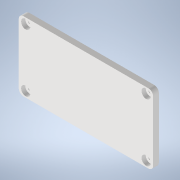
# Autodesk Inventor part: lID
Saved by Autodesk Inventor 2022 (Build 260153000, 153)
## iProperties
Created: 2021-11-08
Part Number: lID
Material: Generisch
Document SubType Name: Modeling
Designer: lukas
Density: 1 g/cm^3
Appearance: Vorgabe
Author: lukas
Autodesk Inventor part; units mm, degrees
ref_plane "YZ Plane" through (0, 0, 0) normal (1, 0, 0) x (0, 1, 0)
ref_plane "XZ Plane" through (0, 0, 0) normal (0, 1, 0) x (-1, 0, 0)
ref_plane "XY Plane" through (0, 0, 0) normal (0, 0, 1) x (1, 0, 0)
sketch "Skizze1" plane through (0, 0, 0) normal (0, 0, 1) x (1, 0, 0)
  arc A0 (-27, 15) -> (-29, 13) centre (-27, 13) ccw projected
  line L0 (-29, 13) -> (-29, 6.9165) projected
  line L1 (-29, 6.9165) -> (-27, 6.9165) projected
  line L2 (-27, 6.9165) -> (-27, 10) projected
  line L3 (-27, 10) -> (-23, 10) projected
  line L4 (-23, 13) -> (-23, 10) projected
  line L5 (-23, 13) -> (23, 13) projected
  line L6 (23, 10) -> (23, 13) projected
  line L7 (27, 10) -> (23, 10) projected
  line L8 (27, 10) -> (27, -10) projected
  line L9 (27, -10) -> (23, -10) projected
  line L10 (23, -13) -> (23, -10) projected
  line L11 (23, -13) -> (-23, -13) projected
  line L12 (-23, -10) -> (-23, -13) projected
  line L13 (-27, -10) -> (-23, -10) projected
  line L14 (-27, -10) -> (-27, -6.9165) projected
  line L15 (-27, -6.9165) -> (-29, -6.9165) projected
  line L16 (-29, -6.9165) -> (-29, -13) projected
  arc A1 (-29, -13) -> (-27, -15) centre (-27, -13) ccw projected
  line L17 (-27, -15) -> (27, -15) projected
  arc A2 (27, -15) -> (29, -13) centre (27, -13) ccw projected
  line L18 (29, -13) -> (29, 13) projected
  arc A3 (29, 13) -> (27, 15) centre (27, 13) ccw projected
  line L19 (27, 15) -> (-27, 15) projected
  circle A4 centre (26, -12.5) radius 1.6 projected
  circle A5 centre (-26, -12.5) radius 1.6 projected
  circle A6 centre (26, 12.5) radius 1.6 projected
  circle A7 centre (-26, 12.5) radius 1.6 projected
  line L20 (-29, 6.9165) -> (-29, -6.9165)
  point P0 (0, 0)
  constraints: 2 end point, 1 collinear
extrude "Extrusion1" add sketch "Skizze1" along normal blind 2.5 contours L19 A3 L18 A2 L17 A1 L16 L15 L14 L13 L12 L11 L10 L9 L8 L7 L6 L5 L4 L3 L2 L1 L0 A0 | L1 L2 L3 L4 L5 L6 L7 L8 L9 L10 L11 L12 L13 L14 L15 L20 | A4 | A5 | A6 | A7
sketch "Skizze2" plane through (0, 0, 2.5) normal (0, 0, 1) x (1, 0, 0)
  circle A0 centre (26, 12.5) radius 1.6 projected
  circle A1 centre (26, -12.5) radius 1.6 projected
  circle A2 centre (-26, -12.5) radius 1.6 projected
  circle A3 centre (-26, 12.5) radius 1.6 projected
  point P0 (0, 0)
hole "Bohrung1" at (-26, -12.5, 2.5) at (-26, 12.5, 2.5) at (26, 12.5, 2.5) at (26, -12.5, 2.5) direction (0, 0, -1) diameter 1.85 end through all counterbore diameter 4 counterbore depth 1.8
sketch "Skizze3" plane through (0, 0, 0) normal (0, 0, -1) x (-1, 0, 0)
  line L0 (12, -13) -> (23, -13) projected
  line L1 (-13, -13) -> (12, -13) projected
  line L2 (-23, -13) -> (-13, -13) projected
  line L3 (23, 13) -> (-23, 13) projected
  line L4 (27, 6.9165) -> (27, 10) projected
  line L5 (27, -10) -> (27, -6.9165) projected
  line L6 (23, -10) -> (23, -13) projected
  line L7 (27, -10) -> (23, -10) projected
  line L8 (-23, -13) -> (-23, -10) projected
  line L9 (-27, -10) -> (-23, -10) projected
  line L10 (23, 13) -> (23, 10) projected
  line L11 (27, 10) -> (23, 10) projected
  line L12 (-23, 10) -> (-23, 13) projected
  line L13 (-27, 10) -> (-23, 10) projected
  line L14 (-27, 10) -> (-27, -10) projected
  line L15 (26.85, 6.9165) -> (26.85, 9.85)
  line L16 (26.85, 9.85) -> (22.85, 9.85)
  line L17 (22.85, 9.85) -> (22.85, 12.85)
  line L18 (22.85, 12.85) -> (-22.85, 12.85)
  line L19 (-22.85, 12.85) -> (-22.85, 9.85)
  line L20 (-22.85, 9.85) -> (-26.85, 9.85)
  line L21 (-26.85, 9.85) -> (-26.85, -9.85)
  line L22 (-26.85, -9.85) -> (-22.85, -9.85)
  line L23 (-22.85, -9.85) -> (-22.85, -12.85)
  line L24 (-22.85, -12.85) -> (-13, -12.85)
  line L25 (-13, -12.85) -> (12, -12.85)
  line L26 (12, -12.85) -> (22.85, -12.85)
  line L27 (22.85, -12.85) -> (22.85, -9.85)
  line L28 (22.85, -9.85) -> (26.85, -9.85)
  line L29 (26.85, -9.85) -> (26.85, -6.9165)
  line L30 (25.85, -6.9165) -> (25.85, -8.85)
  line L31 (25.85, -8.85) -> (21.85, -8.85)
  line L32 (21.85, -8.85) -> (21.85, -11.85)
  line L33 (21.85, -11.85) -> (12, -11.85)
  line L34 (12, -11.85) -> (-13, -11.85)
  line L35 (-13, -11.85) -> (-21.85, -11.85)
  line L36 (-21.85, -11.85) -> (-21.85, -8.85)
  line L37 (-21.85, -8.85) -> (-25.85, -8.85)
  line L38 (-25.85, -8.85) -> (-25.85, 8.85)
  line L39 (-25.85, 8.85) -> (-21.85, 8.85)
  line L40 (-21.85, 8.85) -> (-21.85, 11.85)
  line L41 (-21.85, 11.85) -> (21.85, 11.85)
  line L42 (21.85, 11.85) -> (21.85, 8.85)
  line L43 (21.85, 8.85) -> (25.85, 8.85)
  line L44 (25.85, 8.85) -> (25.85, 6.9165)
  line L45 (26.85, -7.4165) -> (25.8168, -7.4165)
  line L46 (26.85, 7.4165) -> (25.85, 7.4165)
  point P0 (0, 0)
  point P1 (25.85, -7.4165)
  dimension "d9" = 0.15
  dimension "d10" = 1
  dimension "d11" = 0.5
  dimension "d12" = 0.5
  constraints: 64 end point, 3 point on line, 2 horizontal alignment, 2 perpendicular, 28 other
  measures "d9" distance between parallel lines of L7 L28
  measures "d10" distance between parallel lines of L26 L33
  measures "d11" distance from line of L44.end L46
  measures "d12" distance from line of L30.start L45
extrude "Extrusion2" add sketch "Skizze3" along normal blind 1
